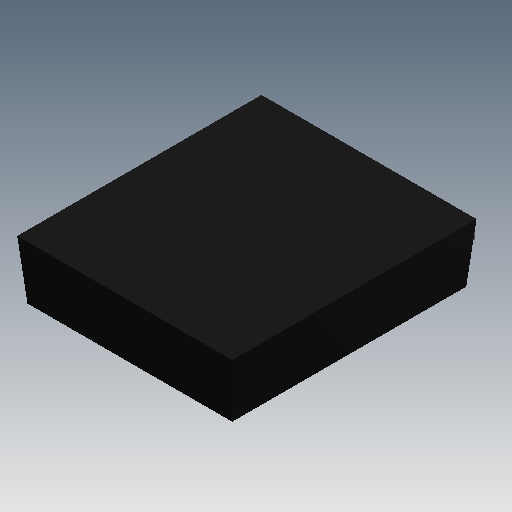
# Autodesk Inventor part: config - chip stand
Saved by Autodesk Inventor 2020 (Build 240152000, 152)
## iProperties
Created: 2005-12-12
Part Number: config - chip stand
Document SubType Name: Modeling
Designer: Simon.Ng@autodesk.com
Stock Number: config - chip stand
Density: 1 g/cm^3
Material: Generic
Mass: 0.1184 g
Surface Area: 1.85413 cm^2
Volume: 0.1184 cm^3
Appearance: Default
Company: Autodesk Asia Pte. Ltd.
Title: PC Demo
Author: Simon.Ng@autodesk.com
Autodesk Inventor part; units mm, degrees
ref_plane "YZ Plane" through (0, 0, 0) normal (1, 0, 0) x (0, 1, 0)
ref_plane "XZ Plane" through (0, 0, 0) normal (0, 1, 0) x (-1, 0, 0)
ref_plane "XY Plane" through (0, 0, 0) normal (0, 0, 1) x (1, 0, 0)
sketch "Sketch2" plane through (0, 0, 0) normal (0, 1, 0) x (-1, 0, 0)
  line L0 (0, -0.1) -> (0, 1.3) projected
  line L1 (-4.8, 0) -> (3.6, 0) projected
  line L2 (-0.5, 0) -> (0.5, 0)
  line L3 (0.5, 0) -> (0.5, 1)
  line L4 (0.5, 1) -> (-0.5, 1)
  line L5 (-0.5, 1) -> (-0.5, 0)
  line L6 (2, 0) -> (3, 0)
  line L7 (3, 0) -> (3, 1)
  line L8 (3, 1) -> (2, 1)
  line L9 (2, 1) -> (2, 0)
  line L10 (-2, 0) -> (-3, 0)
  line L11 (-3, 0) -> (-3, 1)
  line L12 (-3, 1) -> (-2, 1)
  line L13 (-2, 1) -> (-2, 0)
  dimension "d0" = 6
  dimension "d1" = 1
  dimension "d2" = 1
  constraints: 24 end point, 6 parallel, 4 equal length, 3 horizontal, 3 perpendicular, 3 point on line, 2 other
  measures "d0" distance between parallel lines of L11 L7
  measures "d1" distance of L11.end L12.end
  measures "d2" distance of L10.end L11.end
extrude "Extrusion1" add sketch "Sketch2" along normal mid plane 0.5
sketch "Sketch3" plane through (0, 0, 0) normal (0, 1, 0) x (-1, 0, 0)
  line L0 (0, -1.18) -> (0, 15.34) projected
  line L1 (-0.5, 1) -> (0.5, 1) projected
  line L2 (-3.5, 8.8) -> (3.5, 8.8)
  line L3 (3.5, 8.8) -> (3.5, 0.8)
  line L4 (3.5, 0.8) -> (-3.5, 0.8)
  line L5 (-3.5, 0.8) -> (-3.5, 8.8)
  point P0 (0, 0)
  dimension "d5" = 0.2
  dimension "d6" = 8
  dimension "d7" = 7
  constraints: 8 end point, 2 parallel, 1 horizontal, 1 perpendicular, 1 other
  measures "d5" distance between parallel lines of L1 L4
  measures "d6" distance of L4.end L2.start
  measures "d7" distance of L2.start L2.end
extrude "Extrusion2" add sketch "Sketch3" along normal mid plane 2
draft "FaceDraft1" angle 5 pull direction (0, -1, 0) faces at (3.5, 0.3333, 6.1333) (-0.1667, 0.75, 0.8) (-3.5, -0.3333, 6.1333) (-1.1667, 0.3333, 8.8) fixed edges at (3.5, -1, 4.8) (0, -1, 0.8) (-3.5, -1, 4.8) (0, -1, 8.8)
body "Solid1"
